Autodesk Fusion 360 part; units mm, degrees
(part 2 of 9)
  spline S7 degree 5 poles (-8.2602, -45.0085) (-8.2574, -44.9998) (-8.2518, -44.9823) (-8.2434, -44.9561) (-8.2325, -44.9211) (-8.2192, -44.8775) (-8.2062, -44.8338) (-8.1934, -44.7902) (-8.181, -44.7465) (-8.1689, -44.7029) (-8.1571, -44.6593) (-8.1456, -44.6157) (-8.1344, -44.5722) (-8.1235, -44.5286) (-8.1129, -44.4851) (-8.1026, -44.4416) (-8.0927, -44.3982) (-8.083, -44.3547) (-8.0737, -44.3113) (-8.0647, -44.268) (-8.056, -44.2247) (-8.0476, -44.1814) (-8.0396, -44.1381) (-8.0318, -44.0949) (-8.0244, -44.0518) (-8.0174, -44.0087) (-8.0106, -43.9656) (-8.0042, -43.9226) (-7.9981, -43.8797) (-7.9923, -43.8368) (-7.9869, -43.794) (-7.9818, -43.7512) (-7.9771, -43.7085) (-7.9727, -43.6659) (-7.9686, -43.6233) (-7.9649, -43.5808) (-7.9616, -43.5384) (-7.9585, -43.4961) (-7.9559, -43.4538) (-7.9536, -43.4116) (-7.9516, -43.3695) (-7.9501, -43.3275) (-7.9489, -43.2857) (-7.948, -43.2439) (-7.9476, -43.2022) (-7.9475, -43.1606) (-7.9478, -43.1191) (-7.9485, -43.0777) (-7.9495, -43.0364) (-7.951, -42.9953) (-7.9528, -42.9542) (-7.9551, -42.9133) (-7.9578, -42.8726) (-7.961, -42.832) (-7.9646, -42.7915) (-7.9686, -42.7512) (-7.9731, -42.7111) (-7.9779, -42.671) (-7.9831, -42.6312) (-7.9888, -42.5915) (-7.995, -42.552) (-8.0019, -42.5127) (-8.0095, -42.4737) (-8.0177, -42.435) (-8.0265, -42.3965) (-8.0358, -42.3583) (-8.0454, -42.3202) (-8.0554, -42.2822) (-8.0658, -42.2445) (-8.077, -42.2071) (-8.0895, -42.1703) (-8.1011, -42.1416) (-8.1108, -42.1205) (-8.1177, -42.1066) (-8.1213, -42.0998) knots -1 -1 -1 -1 -1 -1 -0.98571429 -0.97142857 -0.95714286 -0.94285714 -0.92857143 -0.91428571 -0.9 -0.88571429 -0.87142857 -0.85714286 -0.84285714 -0.82857143 -0.81428571 -0.8 -0.78571429 -0.77142857 -0.75714286 -0.74285714 -0.72857143 -0.71428571 -0.7 -0.68571429 -0.67142857 -0.65714286 -0.64285714 -0.62857143 -0.61428571 -0.6 -0.58571429 -0.57142857 -0.55714286 -0.54285714 -0.52857143 -0.51428571 -0.5 -0.48571429 -0.47142857 -0.45714286 -0.44285714 -0.42857143 -0.41428571 -0.4 -0.38571429 -0.37142857 -0.35714286 -0.34285714 -0.32857143 -0.31428571 -0.3 -0.28571429 -0.27142857 -0.25714286 -0.24285714 -0.22857143 -0.21428571 -0.2 -0.18571429 -0.17142857 -0.15714286 -0.14285714 -0.12857143 -0.11428571 -0.1 -0.08571429 -0.07142857 -0.05714286 -0.04285714 -0.02857143 -0.01428571 0 0 0 0 0 0
  line L7 (-8.1213, -42.0998) -> (-8.7529, -40.891)
  arc A15 (-8.5688, -40.2318) -> (-8.7529, -40.891) centre (-8.3098, -40.6595) ccw
  arc A16 (-8.5688, -40.2318) -> (-7.5487, -39.4906) centre (-12.4806, -33.7751) ccw
  arc A17 (-6.8649, -39.5193) -> (-7.5487, -39.4906) centre (-7.222, -39.8692) ccw
  line L8 (-6.8649, -39.5193) -> (-5.9105, -40.4935)
  spline S8 degree 5 poles (-5.9105, -40.4935) (-5.905, -40.499) (-5.894, -40.5099) (-5.8769, -40.5256) (-5.8532, -40.5455) (-5.8221, -40.5688) (-5.79, -40.591) (-5.7573, -40.6126) (-5.7243, -40.6338) (-5.691, -40.6547) (-5.6575, -40.6754) (-5.6236, -40.6956) (-5.5894, -40.7154) (-5.5546, -40.7347) (-5.5194, -40.7533) (-5.4838, -40.7714) (-5.4478, -40.7891) (-5.4115, -40.8064) (-5.3749, -40.8234) (-5.338, -40.84) (-5.301, -40.8563) (-5.2636, -40.8722) (-5.226, -40.8878) (-5.1881, -40.903) (-5.1499, -40.9178) (-5.1114, -40.9322) (-5.0728, -40.9463) (-5.0338, -40.9601) (-4.9947, -40.9735) (-4.9553, -40.9866) (-4.9157, -40.9994) (-4.8759, -41.0118) (-4.8359, -41.024) (-4.7957, -41.0358) (-4.7553, -41.0472) (-4.7146, -41.0584) (-4.6738, -41.0692) (-4.6328, -41.0798) (-4.5916, -41.09) (-4.5502, -41.0999) (-4.5087, -41.1095) (-4.4669, -41.1188) (-4.425, -41.1278) (-4.383, -41.1365) (-4.3407, -41.1449) (-4.2983, -41.1529) (-4.2557, -41.1607) (-4.213, -41.1682) (-4.1701, -41.1754) (-4.1271, -41.1823) (-4.0839, -41.1888) (-4.0406, -41.1951) (-3.9971, -41.2011) (-3.9535, -41.2068) (-3.9098, -41.2122) (-3.8659, -41.2174) (-3.8218, -41.2222) (-3.7777, -41.2267) (-3.7334, -41.231) (-3.689, -41.2349) (-3.6445, -41.2386) (-3.5998, -41.242) (-3.555, -41.2451) (-3.5102, -41.2479) (-3.4651, -41.2504) (-3.42, -41.2527) (-3.3748, -41.2546) (-3.3295, -41.2563) (-3.284, -41.2576) (-3.2385, -41.2587) (-3.1928, -41.2596) (-3.1562, -41.26) (-3.1287, -41.2602) (-3.1104, -41.2602) (-3.1012, -41.2603) knots 0 0 0 0 0 0 0.01428571 0.02857143 0.04285714 0.05714286 0.07142857 0.08571429 0.1 0.11428571 0.12857143 0.14285714 0.15714286 0.17142857 0.18571429 0.2 0.21428571 0.22857143 0.24285714 0.25714286 0.27142857 0.28571429 0.3 0.31428571 0.32857143 0.34285714 0.35714286 0.37142857 0.38571429 0.4 0.41428571 0.42857143 0.44285714 0.45714286 0.47142857 0.48571429 0.5 0.51428571 0.52857143 0.54285714 0.55714286 0.57142857 0.58571429 0.6 0.61428571 0.62857143 0.64285714 0.65714286 0.67142857 0.68571429 0.7 0.71428571 0.72857143 0.74285714 0.75714286 0.77142857 0.78571429 0.8 0.81428571 0.82857143 0.84285714 0.85714286 0.87142857 0.88571429 0.9 0.91428571 0.92857143 0.94285714 0.95714286 0.97142857 0.98571429 1 1 1 1 1 1
  arc A18 (-3.1012, -41.2603) -> (-2.4634, -40.3824) centre (-12.4806, -33.7751) ccw
  spline S9 degree 5 poles (-2.4634, -40.3824) (-2.4663, -40.3737) (-2.472, -40.3563) (-2.4807, -40.3302) (-2.4924, -40.2955) (-2.5073, -40.2523) (-2.5224, -40.2094) (-2.5377, -40.1666) (-2.5533, -40.124) (-2.5692, -40.0816) (-2.5852, -40.0393) (-2.6015, -39.9973) (-2.6181, -39.9555) (-2.6349, -39.9139) (-2.6519, -39.8724) (-2.6691, -39.8312) (-2.6866, -39.7902) (-2.7043, -39.7494) (-2.7223, -39.7088) (-2.7405, -39.6684) (-2.7589, -39.6283) (-2.7776, -39.5883) (-2.7965, -39.5486) (-2.8156, -39.5091) (-2.835, -39.4699) (-2.8546, -39.4308) (-2.8745, -39.392) (-2.8945, -39.3535) (-2.9149, -39.3152) (-2.9354, -39.2771) (-2.9562, -39.2392) (-2.9772, -39.2017) (-2.9985, -39.1643) (-3.02, -39.1272) (-3.0417, -39.0904) (-3.0637, -39.0539) (-3.0859, -39.0176) (-3.1084, -38.9816) (-3.131, -38.9458) (-3.154, -38.9103) (-3.1771, -38.8751) (-3.2005, -38.8402) (-3.2242, -38.8056) (-3.2481, -38.7713) (-3.2722, -38.7373) (-3.2966, -38.7036) (-3.3213, -38.6702) (-3.3461, -38.6372) (-3.3712, -38.6044) (-3.3966, -38.5719) (-3.4222, -38.5398) (-3.4481, -38.5081) (-3.4742, -38.4767) (-3.5007, -38.4458) (-3.5274, -38.4152) (-3.5543, -38.3849) (-3.5815, -38.355) (-3.609, -38.3255) (-3.6366, -38.2963) (-3.6646, -38.2675) (-3.6928, -38.2392) (-3.7215, -38.2115) (-3.7505, -38.1844) (-3.7799, -38.1579) (-3.8096, -38.132) (-3.8396, -38.1065) (-3.8698, -38.0813) (-3.9002, -38.0564) (-3.9308, -38.032) (-3.9618, -38.0084) (-3.9936, -37.986) (-4.0198, -37.9696) (-4.0401, -37.9582) (-4.0538, -37.9511) (-4.0608, -37.9476) knots -1 -1 -1 -1 -1 -1 -0.98571429 -0.97142857 -0.95714286 -0.94285714 -0.92857143 -0.91428571 -0.9 -0.88571429 -0.87142857 -0.85714286 -0.84285714 -0.82857143 -0.81428571 -0.8 -0.78571429 -0.77142857 -0.75714286 -0.74285714 -0.72857143 -0.71428571 -0.7 -0.68571429 -0.67142857 -0.65714286 -0.64285714 -0.62857143 -0.61428571 -0.6 -0.58571429 -0.57142857 -0.55714286 -0.54285714 -0.52857143 -0.51428571 -0.5 -0.48571429 -0.47142857 -0.45714286 -0.44285714 -0.42857143 -0.41428571 -0.4 -0.38571429 -0.37142857 -0.35714286 -0.34285714 -0.32857143 -0.31428571 -0.3 -0.28571429 -0.27142857 -0.25714286 -0.24285714 -0.22857143 -0.21428571 -0.2 -0.18571429 -0.17142857 -0.15714286 -0.14285714 -0.12857143 -0.11428571 -0.1 -0.08571429 -0.07142857 -0.05714286 -0.04285714 -0.02857143 -0.01428571 0 0 0 0 0 0
  line L9 (-4.0608, -37.9476) -> (-5.2822, -37.341)
  arc A19 (-5.5208, -36.6995) -> (-5.2822, -37.341) centre (-5.0598, -36.8932) ccw
  arc A20 (-5.5208, -36.6995) -> (-5.1311, -35.5002) centre (-12.4806, -33.7751) ccw
  arc A21 (-4.561, -35.1214) -> (-5.1311, -35.5002) centre (-4.6443, -35.6144) ccw
  line L10 (-4.561, -35.1214) -> (-3.2163, -35.3486)
  spline S10 degree 5 poles (-3.2163, -35.3486) (-3.2087, -35.3499) (-3.1933, -35.3522) (-3.1703, -35.3549) (-3.1394, -35.357) (-3.1005, -35.3576) (-3.0615, -35.3567) (-3.0224, -35.3549) (-2.9832, -35.3527) (-2.944, -35.35) (-2.9048, -35.347) (-2.8654, -35.3435) (-2.8261, -35.3394) (-2.7867, -35.3345) (-2.7472, -35.3289) (-2.7077, -35.3227) (-2.6682, -35.3158) (-2.6287, -35.3085) (-2.5891, -35.3007) (-2.5495, -35.2925) (-2.51, -35.2838) (-2.4704, -35.2748) (-2.4308, -35.2653) (-2.3912, -35.2553) (-2.3516, -35.2448) (-2.312, -35.2339) (-2.2724, -35.2225) (-2.2328, -35.2108) (-2.1933, -35.1986) (-2.1537, -35.1861) (-2.1142, -35.1732) (-2.0747, -35.1599) (-2.0352, -35.1462) (-1.9957, -35.1321) (-1.9562, -35.1176) (-1.9168, -35.1027) (-1.8774, -35.0875) (-1.838, -35.0719) (-1.7987, -35.056) (-1.7594, -35.0397) (-1.7201, -35.023) (-1.6809, -35.006) (-1.6417, -34.9886) (-1.6026, -34.9709) (-1.5635, -34.9529) (-1.5244, -34.9345) (-1.4854, -34.9158) (-1.4464, -34.8967) (-1.4075, -34.8773) (-1.3687, -34.8576) (-1.3299, -34.8375) (-1.2911, -34.8171) (-1.2524, -34.7964) (-1.2138, -34.7754) (-1.1752, -34.7541) (-1.1367, -34.7324) (-1.0982, -34.7105) (-1.0599, -34.6882) (-1.0215, -34.6656) (-0.9833, -34.6427) (-0.9451, -34.6195) (-0.907, -34.596) (-0.8689, -34.5722) (-0.831, -34.548) (-0.7931, -34.5236) (-0.7553, -34.4989) (-0.7175, -34.4739) (-0.6799, -34.4486) (-0.6423, -34.423) (-0.6048, -34.3971) (-0.5674, -34.371) (-0.5375, -34.3498) (-0.5152, -34.3338) (-0.5003, -34.3231) (-0.4928, -34.3177) knots 0 0 0 0 0 0 0.01428571 0.02857143 0.04285714 0.05714286 0.07142857 0.08571429 0.1 0.11428571 0.12857143 0.14285714 0.15714286 0.17142857 0.18571429 0.2 0.21428571 0.22857143 0.24285714 0.25714286 0.27142857 0.28571429 0.3 0.31428571 0.32857143 0.34285714 0.35714286 0.37142857 0.38571429 0.4 0.41428571 0.42857143 0.44285714 0.45714286 0.47142857 0.48571429 0.5 0.51428571 0.52857143 0.54285714 0.55714286 0.57142857 0.58571429 0.6 0.61428571 0.62857143 0.64285714 0.65714286 0.67142857 0.68571429 0.7 0.71428571 0.72857143 0.74285714 0.75714286 0.77142857 0.78571429 0.8 0.81428571 0.82857143 0.84285714 0.85714286 0.87142857 0.88571429 0.9 0.91428571 0.92857143 0.94285714 0.95714286 0.97142857 0.98571429 1 1 1 1 1 1
  arc A22 (-0.4928, -34.3177) -> (-0.4928, -33.2326) centre (-12.4806, -33.7751) ccw
  spline S11 degree 5 poles (-0.4928, -33.2326) (-0.5003, -33.2272) (-0.5152, -33.2165) (-0.5375, -33.2005) (-0.5674, -33.1793) (-0.6048, -33.1532) (-0.6423, -33.1273) (-0.6799, -33.1017) (-0.7175, -33.0764) (-0.7553, -33.0514) (-0.7931, -33.0267) (-0.831, -33.0022) (-0.8689, -32.9781) (-0.907, -32.9543) (-0.9451, -32.9308) (-0.9833, -32.9076) (-1.0215, -32.8847) (-1.0599, -32.8621) (-1.0982, -32.8398) (-1.1367, -32.8179) (-1.1752, -32.7962) (-1.2138, -32.7749) (-1.2524, -32.7538) (-1.2911, -32.7331) (-1.3299, -32.7128) (-1.3687, -32.6927) (-1.4075, -32.673) (-1.4464, -32.6536) (-1.4854, -32.6345) (-1.5244, -32.6158) (-1.5635, -32.5974) (-1.6026, -32.5794) (-1.6417, -32.5617) (-1.6809, -32.5443) (-1.7201, -32.5273) (-1.7594, -32.5106) (-1.7987, -32.4943) (-1.838, -32.4784) (-1.8774, -32.4628) (-1.9168, -32.4476) (-1.9562, -32.4327) (-1.9957, -32.4182) (-2.0352, -32.4041) (-2.0747, -32.3904) (-2.1142, -32.3771) (-2.1537, -32.3642) (-2.1933, -32.3517) (-2.2328, -32.3395) (-2.2724, -32.3277) (-2.312, -32.3164) (-2.3516, -32.3055) (-2.3912, -32.295) (-2.4308, -32.285) (-2.4704, -32.2755) (-2.51, -32.2664) (-2.5495, -32.2578) (-2.5891, -32.2496) (-2.6287, -32.2418) (-2.6682, -32.2345) (-2.7077, -32.2276) (-2.7472, -32.2213) (-2.7867, -32.2157) (-2.8261, -32.2109) (-2.8654, -32.2067) (-2.9048, -32.2033) (-2.944, -32.2003) (-2.9832, -32.1976) (-3.0224, -32.1954) (-3.0615, -32.1936) (-3.1005, -32.1927) (-3.1394, -32.1933) (-3.1703, -32.1954) (-3.1933, -32.1981) (-3.2087, -32.2004) (-3.2163, -32.2017) knots -1 -1 -1 -1 -1 -1 -0.98571429 -0.97142857 -0.95714286 -0.94285714 -0.92857143 -0.91428571 -0.9 -0.88571429 -0.87142857 -0.85714286 -0.84285714 -0.82857143 -0.81428571 -0.8 -0.78571429 -0.77142857 -0.75714286 -0.74285714 -0.72857143 -0.71428571 -0.7 -0.68571429 -0.67142857 -0.65714286 -0.64285714 -0.62857143 -0.61428571 -0.6 -0.58571429 -0.57142857 -0.55714286 -0.54285714 -0.52857143 -0.51428571 -0.5 -0.48571429 -0.47142857 -0.45714286 -0.44285714 -0.42857143 -0.41428571 -0.4 -0.38571429 -0.37142857 -0.35714286 -0.34285714 -0.32857143 -0.31428571 -0.3 -0.28571429 -0.27142857 -0.25714286 -0.24285714 -0.22857143 -0.21428571 -0.2 -0.18571429 -0.17142857 -0.15714286 -0.14285714 -0.12857143 -0.11428571 -0.1 -0.08571429 -0.07142857 -0.05714286 -0.04285714 -0.02857143 -0.01428571 0 0 0 0 0 0
  line L11 (-3.2163, -32.2017) -> (-4.561, -32.4289)
  arc A23 (-5.1311, -32.0501) -> (-4.561, -32.4289) centre (-4.6443, -31.9359) ccw
  arc A24 (-5.1311, -32.0501) -> (-5.5208, -30.8508) centre (-12.4806, -33.7751) ccw
  arc A25 (-5.2822, -30.2093) -> (-5.5208, -30.8508) centre (-5.0598, -30.6571) ccw
  line L12 (-5.2822, -30.2093) -> (-4.0608, -29.6027)
  spline S12 degree 5 poles (-4.0608, -29.6027) (-4.0538, -29.5992) (-4.0401, -29.5921) (-4.0198, -29.5807) (-3.9936, -29.5643) (-3.9618, -29.5419) (-3.9308, -29.5183) (-3.9002, -29.4939) (-3.8698, -29.469) (-3.8396, -29.4438) (-3.8096, -29.4183) (-3.7799, -29.3924) (-3.7505, -29.3659) (-3.7215, -29.3388) (-3.6928, -29.3111) (-3.6646, -29.2828) (-3.6366, -29.254) (-3.609, -29.2248) (-3.5815, -29.1953) (-3.5543, -29.1654) (-3.5274, -29.1351) (-3.5007, -29.1045) (-3.4742, -29.0736) (-3.4481, -29.0422) (-3.4222, -29.0105) (-3.3966, -28.9784) (-3.3712, -28.9459) (-3.3461, -28.9131) (-3.3213, -28.8801) (-3.2966, -28.8467) (-3.2722, -28.813) (-3.2481, -28.779) (-3.2242, -28.7447) (-3.2005, -28.7101) (-3.1771, -28.6752) (-3.154, -28.64) (-3.131, -28.6045) (-3.1084, -28.5687) (-3.0859, -28.5327) (-3.0637, -28.4964) (-3.0417, -28.4599) (-3.02, -28.423) (-2.9985, -28.386) (-2.9772, -28.3486) (-2.9562, -28.311) (-2.9354, -28.2732) (-2.9149, -28.2351) (-2.8945, -28.1968) (-2.8745, -28.1582) (-2.8546, -28.1194) (-2.835, -28.0804) (-2.8156, -28.0411) (-2.7965, -28.0017) (-2.7776, -27.9619) (-2.7589, -27.922) (-2.7405, -27.8818) (-2.7223, -27.8415) (-2.7043, -27.8009) (-2.6866, -27.7601) (-2.6691, -27.7191) (-2.6519, -27.6779) (-2.6349, -27.6364) (-2.6181, -27.5948) (-2.6015, -27.553) (-2.5852, -27.511) (-2.5692, -27.4687) (-2.5533, -27.4263) (-2.5377, -27.3837) (-2.5224, -27.3409) (-2.5073, -27.2979) (-2.4924, -27.2548) (-2.4807, -27.2201) (-2.472, -27.194) (-2.4663, -27.1766) (-2.4634, -27.1678) knots 0 0 0 0 0 0 0.01428571 0.02857143 0.04285714 0.05714286 0.07142857 0.08571429 0.1 0.11428571 0.12857143 0.14285714 0.15714286 0.17142857 0.18571429 0.2 0.21428571 0.22857143 0.24285714 0.25714286 0.27142857 0.28571429 0.3 0.31428571 0.32857143 0.34285714 0.35714286 0.37142857 0.38571429 0.4 0.41428571 0.42857143 0.44285714 0.45714286 0.47142857 0.48571429 0.5 0.51428571 0.52857143 0.54285714 0.55714286 0.57142857 0.58571429 0.6 0.61428571 0.62857143 0.64285714 0.65714286 0.67142857 0.68571429 0.7 0.71428571 0.72857143 0.74285714 0.75714286 0.77142857 0.78571429 0.8 0.81428571 0.82857143 0.84285714 0.85714286 0.87142857 0.88571429 0.9 0.91428571 0.92857143 0.94285714 0.95714286 0.97142857 0.98571429 1 1 1 1 1 1
  arc A26 (-2.4634, -27.1678) -> (-3.1012, -26.29) centre (-12.4806, -33.7751) ccw
  spline S13 degree 5 poles (-3.1012, -26.29) (-3.1104, -26.29) (-3.1287, -26.2901) (-3.1562, -26.2903) (-3.1928, -26.2907) (-3.2385, -26.2915) (-3.284, -26.2926) (-3.3295, -26.294) (-3.3748, -26.2957) (-3.42, -26.2976) (-3.4651, -26.2999) (-3.5102, -26.3024) (-3.555, -26.3052) (-3.5998, -26.3083) (-3.6445, -26.3117) (-3.689, -26.3153) (-3.7334, -26.3193) (-3.7777, -26.3236) (-3.8218, -26.3281) (-3.8659, -26.3329) (-3.9098, -26.338) (-3.9535, -26.3435) (-3.9971, -26.3492) (-4.0406, -26.3552) (-4.0839, -26.3614) (-4.1271, -26.368) (-4.1701, -26.3749) (-4.213, -26.3821) (-4.2557, -26.3896) (-4.2983, -26.3974) (-4.3407, -26.4054) (-4.383, -26.4138) (-4.425, -26.4225) (-4.4669, -26.4315) (-4.5087, -26.4408) (-4.5502, -26.4504) (-4.5916, -26.4603) (-4.6328, -26.4705) (-4.6738, -26.481) (-4.7146, -26.4919) (-4.7553, -26.503) (-4.7957, -26.5145) (-4.8359, -26.5263) (-4.8759, -26.5384) (-4.9157, -26.5509) (-4.9553, -26.5637) (-4.9947, -26.5768) (-5.0338, -26.5902) (-5.0728, -26.604) (-5.1114, -26.6181) (-5.1499, -26.6325) (-5.1881, -26.6473) (-5.226, -26.6625) (-5.2636, -26.6781) (-5.301, -26.694) (-5.338, -26.7103) (-5.3749, -26.7269) (-5.4115, -26.7439) (-5.4478, -26.7612) (-5.4838, -26.7788) (-5.5194, -26.797) (-5.5546, -26.8156) (-5.5894, -26.8349) (-5.6236, -26.8547) (-5.6575, -26.8749) (-5.691, -26.8956) (-5.7243, -26.9165) (-5.7573, -26.9377) (-5.79, -26.9592) (-5.8221, -26.9815) (-5.8532, -27.0048) (-5.8769, -27.0246) (-5.894, -27.0404) (-5.905, -27.0513) (-5.9105, -27.0568) knots -1 -1 -1 -1 -1 -1 -0.98571429 -0.97142857 -0.95714286 -0.94285714 -0.92857143 -0.91428571 -0.9 -0.88571429 -0.87142857 -0.85714286 -0.84285714 -0.82857143 -0.81428571 -0.8 -0.78571429 -0.77142857 -0.75714286 -0.74285714 -0.72857143 -0.71428571 -0.7 -0.68571429 -0.67142857 -0.65714286 -0.64285714 -0.62857143 -0.61428571 -0.6 -0.58571429 -0.57142857 -0.55714286 -0.54285714 -0.52857143 -0.51428571 -0.5 -0.48571429 -0.47142857 -0.45714286 -0.44285714 -0.42857143 -0.41428571 -0.4 -0.38571429 -0.37142857 -0.35714286 -0.34285714 -0.32857143 -0.31428571 -0.3 -0.28571429 -0.27142857 -0.25714286 -0.24285714 -0.22857143 -0.21428571 -0.2 -0.18571429 -0.17142857 -0.15714286 -0.14285714 -0.12857143 -0.11428571 -0.1 -0.08571429 -0.07142857 -0.05714286 -0.04285714 -0.02857143 -0.01428571 0 0 0 0 0 0
  line L13 (-5.9105, -27.0568) -> (-6.8649, -28.031)
  arc A27 (-7.5487, -28.0597) -> (-6.8649, -28.031) centre (-7.222, -27.6811) ccw
  arc A28 (-7.5487, -28.0597) -> (-8.5688, -27.3185) centre (-12.4806, -33.7751) ccw
  arc A29 (-8.7529, -26.6593) -> (-8.5688, -27.3185) centre (-8.3098, -26.8908) ccw
  line L14 (-8.7529, -26.6593) -> (-8.1213, -25.4505)
  spline S14 degree 5 poles (-8.1213, -25.4505) (-8.1177, -25.4437) (-8.1108, -25.4298) (-8.1011, -25.4087) (-8.0895, -25.3799) (-8.077, -25.3432) (-8.0658, -25.3058) (-8.0554, -25.2681) (-8.0454, -25.2301) (-8.0358, -25.192) (-8.0265, -25.1537) (-8.0177, -25.1153) (-8.0095, -25.0766) (-8.0019, -25.0376) (-7.995, -24.9983) (-7.9888, -24.9588) (-7.9831, -24.9191) (-7.9779, -24.8792) (-7.9731, -24.8392) (-7.9686, -24.799) (-7.9646, -24.7587) (-7.961, -24.7183) (-7.9578, -24.6777) (-7.9551, -24.637) (-7.9528, -24.5961) (-7.951, -24.555) (-7.9495, -24.5139) (-7.9485, -24.4726) (-7.9478, -24.4312) (-7.9475, -24.3897) (-7.9476, -24.3481) (-7.948, -24.3064) (-7.9489, -24.2646) (-7.9501, -24.2227) (-7.9516, -24.1807) (-7.9536, -24.1387) (-7.9559, -24.0965) (-7.9585, -24.0542) (-7.9616, -24.0119) (-7.9649, -23.9695) (-7.9686, -23.927) (-7.9727, -23.8844) (-7.9771, -23.8418) (-7.9818, -23.7991) (-7.9869, -23.7563) (-7.9923, -23.7135) (-7.9981, -23.6706) (-8.0042, -23.6276) (-8.0106, -23.5846) (-8.0174, -23.5416) (-8.0244, -23.4985) (-8.0318, -23.4553) (-8.0396, -23.4121) (-8.0476, -23.3689) (-8.056, -23.3256) (-8.0647, -23.2823) (-8.0737, -23.2389) (-8.083, -23.1956) (-8.0927, -23.1521) (-8.1026, -23.1087) (-8.1129, -23.0652) (-8.1235, -23.0217) (-8.1344, -22.9781) (-8.1456, -22.9346) (-8.1571, -22.891) (-8.1689, -22.8474) (-8.181, -22.8038) (-8.1934, -22.7601) (-8.2062, -22.7165) (-8.2192, -22.6728) (-8.2325, -22.6292) (-8.2434, -22.5942) (-8.2518, -22.568) (-8.2574, -22.5505) (-8.2602, -22.5418) knots 0 0 0 0 0 0 0.01428571 0.02857143 0.04285714 0.05714286 0.07142857 0.08571429 0.1 0.11428571 0.12857143 0.14285714 0.15714286 0.17142857 0.18571429 0.2 0.21428571 0.22857143 0.24285714 0.25714286 0.27142857 0.28571429 0.3 0.31428571 0.32857143 0.34285714 0.35714286 0.37142857 0.38571429 0.4 0.41428571 0.42857143 0.44285714 0.45714286 0.47142857 0.48571429 0.5 0.51428571 0.52857143 0.54285714 0.55714286 0.57142857 0.58571429 0.6 0.61428571 0.62857143 0.64285714 0.65714286 0.67142857 0.68571429 0.7 0.71428571 0.72857143 0.74285714 0.75714286 0.77142857 0.78571429 0.8 0.81428571 0.82857143 0.84285714 0.85714286 0.87142857 0.88571429 0.9 0.91428571 0.92857143 0.94285714 0.95714286 0.97142857 0.98571429 1 1 1 1 1 1
  arc A30 (-8.2602, -22.5418) -> (-9.2921, -22.2065) centre (-12.4806, -33.7751) ccw
  spline S15 degree 5 poles (-9.2921, -22.2065) (-9.2995, -22.2119) (-9.3144, -22.2227) (-9.3365, -22.2391) (-9.3658, -22.2609) (-9.4023, -22.2884) (-9.4385, -22.3161) (-9.4745, -22.3439) (-9.5102, -22.3719) (-9.5456, -22.4001) (-9.5808, -22.4284) (-9.6157, -22.4569) (-9.6504, -22.4855) (-9.6848, -22.5144) (-9.7189, -22.5433) (-9.7528, -22.5725) (-9.7864, -22.6018) (-9.8197, -22.6313) (-9.8528, -22.6609) (-9.8856, -22.6907) (-9.9181, -22.7206) (-9.9503, -22.7507) (-9.9822, -22.7809) (-10.0138, -22.8113) (-10.0452, -22.8419) (-10.0763, -22.8726) (-10.107, -22.9035) (-10.1375, -22.9345) (-10.1677, -22.9657) (-10.1975, -22.997) (-10.2271, -23.0284) (-10.2563, -23.06) (-10.2853, -23.0918) (-10.3139, -23.1237) (-10.3422, -23.1558) (-10.3702, -23.188) (-10.3978, -23.2203) (-10.4251, -23.2528) (-10.4521, -23.2854) (-10.4788, -23.3182) (-10.5051, -23.3511) (-10.5311, -23.3841) (-10.5567, -23.4173) (-10.5819, -23.4506) (-10.6068, -23.4841) (-10.6313, -23.5177) (-10.6554, -23.5515) (-10.6792, -23.5853) (-10.7026, -23.6193) (-10.7257, -23.6535) (-10.7483, -23.6878) (-10.7705, -23.7222) (-10.7922, -23.7568) (-10.8135, -23.7915) (-10.8343, -23.8263) (-10.8548, -23.8613) (-10.8748, -23.8964) (-10.8944, -23.9316) (-10.9136, -23.9669) (-10.9324, -24.0024) (-10.9505, -24.038) (-10.9681, -24.0738) (-10.9849, -24.1098) (-11.001, -24.146) (-11.0164, -24.1823) (-11.0314, -24.2187) (-11.046, -24.2552) (-11.0603, -24.2917) (-11.0741, -24.3284) (-11.087, -24.3652) (-11.0984, -24.4023) (-11.106, -24.4323) (-11.1105, -24.4551) (-11.113, -24.4704) (-11.1142, -24.4781) knots -1 -1 -1 -1 -1 -1 -0.98571429 -0.97142857 -0.95714286 -0.94285714 -0.92857143 -0.91428571 -0.9 -0.88571429 -0.87142857 -0.85714286 -0.84285714 -0.82857143 -0.81428571 -0.8 -0.78571429 -0.77142857 -0.75714286 -0.74285714 -0.72857143 -0.71428571 -0.7 -0.68571429 -0.67142857 -0.65714286 -0.64285714 -0.62857143 -0.61428571 -0.6 -0.58571429 -0.57142857 -0.55714286 -0.54285714 -0.52857143 -0.51428571 -0.5 -0.48571429 -0.47142857 -0.45714286 -0.44285714 -0.42857143 -0.41428571 -0.4 -0.38571429 -0.37142857 -0.35714286 -0.34285714 -0.32857143 -0.31428571 -0.3 -0.28571429 -0.27142857 -0.25714286 -0.24285714 -0.22857143 -0.21428571 -0.2 -0.18571429 -0.17142857 -0.15714286 -0.14285714 -0.12857143 -0.11428571 -0.1 -0.08571429 -0.07142857 -0.05714286 -0.04285714 -0.02857143 -0.01428571 0 0 0 0 0 0
  line L15 (-11.1142, -24.4781) -> (-11.3137, -25.8272)
  arc A31 (-11.8501, -26.2523) -> (-11.3137, -25.8272) centre (-11.8083, -25.7541) ccw
  arc A32 (-11.8501, -26.2523) -> (-13.1111, -26.2523) centre (-12.4806, -33.7751) ccw
  arc A33 (-13.6474, -25.8272) -> (-13.1111, -26.2523) centre (-13.1528, -25.7541) ccw
  line L16 (-13.6474, -25.8272) -> (-13.847, -24.4781)
  spline S16 degree 5 poles (-13.847, -24.4781) (-13.8481, -24.4704) (-13.8506, -24.4551) (-13.8552, -24.4323) (-13.8627, -24.4023) (-13.8742, -24.3652) (-13.887, -24.3284) (-13.9008, -24.2917) (-13.9151, -24.2552) (-13.9297, -24.2187) (-13.9447, -24.1823) (-13.9602, -24.146) (-13.9763, -24.1098) (-13.9931, -24.0738) (-14.0106, -24.038) (-14.0288, -24.0024) (-14.0475, -23.9669) (-14.0667, -23.9316) (-14.0863, -23.8964) (-14.1064, -23.8613) (-14.1268, -23.8263) (-14.1476, -23.7915) (-14.1689, -23.7568) (-14.1907, -23.7222) (-14.2129, -23.6878) (-14.2355, -23.6535) (-14.2585, -23.6193) (-14.2819, -23.5853) (-14.3057, -23.5515) (-14.3298, -23.5177) (-14.3544, -23.4841) (-14.3792, -23.4506) (-14.4045, -23.4173) (-14.4301, -23.3841) (-14.456, -23.3511) (-14.4823, -23.3182) (-14.509, -23.2854) (-14.536, -23.2528) (-14.5633, -23.2203) (-14.591, -23.188) (-14.6189, -23.1558) (-14.6472, -23.1237) (-14.6759, -23.0918) (-14.7048, -23.06) (-14.734, -23.0284) (-14.7636, -22.997) (-14.7935, -22.9657) (-14.8236, -22.9345) (-14.8541, -22.9035) (-14.8849, -22.8726) (-14.9159, -22.8419) (-14.9473, -22.8113) (-14.9789, -22.7809) (-15.0109, -22.7507) (-15.0431, -22.7206) (-15.0756, -22.6907) (-15.1084, -22.6609) (-15.1414, -22.6313) (-15.1747, -22.6018) (-15.2083, -22.5725) (-15.2422, -22.5433) (-15.2763, -22.5144) (-15.3107, -22.4855) (-15.3454, -22.4569) (-15.3803, -22.4284) (-15.4155, -22.4001) (-15.451, -22.3719) (-15.4867, -22.3439) (-15.5226, -22.3161) (-15.5588, -22.2884) (-15.5953, -22.2609) (-15.6246, -22.2391) (-15.6468, -22.2227) (-15.6616, -22.2119) (-15.669, -22.2065) knots 0 0 0 0 0 0 0.01428571 0.02857143 0.04285714 0.05714286 0.07142857 0.08571429 0.1 0.11428571 0.12857143 0.14285714 0.15714286 0.17142857 0.18571429 0.2 0.21428571 0.22857143 0.24285714 0.25714286 0.27142857 0.28571429 0.3 0.31428571 0.32857143 0.34285714 0.35714286 0.37142857 0.38571429 0.4 0.41428571 0.42857143 0.44285714 0.45714286 0.47142857 0.48571429 0.5 0.51428571 0.52857143 0.54285714 0.55714286 0.57142857 0.58571429 0.6 0.61428571 0.62857143 0.64285714 0.65714286 0.67142857 0.68571429 0.7 0.71428571 0.72857143 0.74285714 0.75714286 0.77142857 0.78571429 0.8 0.81428571 0.82857143 0.84285714 0.85714286 0.87142857 0.88571429 0.9 0.91428571 0.92857143 0.94285714 0.95714286 0.97142857 0.98571429 1 1 1 1 1 1
  arc A34 (-15.669, -22.2065) -> (-16.701, -22.5418) centre (-12.4806, -33.7751) ccw
  spline S17 degree 5 poles (-16.701, -22.5418) (-16.7038, -22.5505) (-16.7094, -22.568) (-16.7177, -22.5942) (-16.7286, -22.6292) (-16.7419, -22.6728) (-16.755, -22.7165) (-16.7677, -22.7601) (-16.7801, -22.8038) (-16.7922, -22.8474) (-16.8041, -22.891) (-16.8156, -22.9346) (-16.8268, -22.9781) (-16.8377, -23.0217) (-16.8482, -23.0652) (-16.8585, -23.1087) (-16.8685, -23.1521) (-16.8781, -23.1956) (-16.8874, -23.2389) (-16.8965, -23.2823) (-16.9051, -23.3256) (-16.9135, -23.3689) (-16.9216, -23.4121) (-16.9293, -23.4553) (-16.9367, -23.4985) (-16.9438, -23.5416) (-16.9505, -23.5846) (-16.957, -23.6276) (-16.963, -23.6706) (-16.9688, -23.7135) (-16.9742, -23.7563) (-16.9793, -23.7991) (-16.984, -23.8418) (-16.9884, -23.8844) (-16.9925, -23.927) (-16.9962, -23.9695) (-16.9996, -24.0119) (-17.0026, -24.0542) (-17.0053, -24.0965) (-17.0076, -24.1387) (-17.0095, -24.1807) (-17.0111, -24.2227) (-17.0123, -24.2646) (-17.0131, -24.3064) (-17.0136, -24.3481) (-17.0136, -24.3897) (-17.0133, -24.4312) (-17.0127, -24.4726) (-17.0116, -24.5139) (-17.0102, -24.555) (-17.0083, -24.5961) (-17.006, -24.637) (-17.0033, -24.6777) (-17.0001, -24.7183) (-16.9965, -24.7587) (-16.9925, -24.799) (-16.9881, -24.8392) (-16.9832, -24.8792) (-16.978, -24.9191) (-16.9723, -24.9588) (-16.9661, -24.9983) (-16.9592, -25.0376) (-16.9517, -25.0766) (-16.9434, -25.1153) (-16.9346, -25.1537) (-16.9253, -25.192) (-16.9157, -25.2301) (-16.9058, -25.2681) (-16.8954, -25.3058) (-16.8842, -25.3432) (-16.8716, -25.3799) (-16.86, -25.4087) (-16.8503, -25.4298) (-16.8434, -25.4437) (-16.8398, -25.4505) knots -1 -1 -1 -1 -1 -1 -0.98571429 -0.97142857 -0.95714286 -0.94285714 -0.92857143 -0.91428571 -0.9 -0.88571429 -0.87142857 -0.85714286 -0.84285714 -0.82857143 -0.81428571 -0.8 -0.78571429 -0.77142857 -0.75714286 -0.74285714 -0.72857143 -0.71428571 -0.7 -0.68571429 -0.67142857 -0.65714286 -0.64285714 -0.62857143 -0.61428571 -0.6 -0.58571429 -0.57142857 -0.55714286 -0.54285714 -0.52857143 -0.51428571 -0.5 -0.48571429 -0.47142857 -0.45714286 -0.44285714 -0.42857143 -0.41428571 -0.4 -0.38571429 -0.37142857 -0.35714286 -0.34285714 -0.32857143 -0.31428571 -0.3 -0.28571429 -0.27142857 -0.25714286 -0.24285714 -0.22857143 -0.21428571 -0.2 -0.18571429 -0.17142857 -0.15714286 -0.14285714 -0.12857143 -0.11428571 -0.1 -0.08571429 -0.07142857 -0.05714286 -0.04285714 -0.02857143 -0.01428571 0 0 0 0 0 0
  line L17 (-16.8398, -25.4505) -> (-16.2082, -26.6593)
  arc A35 (-16.3923, -27.3185) -> (-16.2082, -26.6593) centre (-16.6514, -26.8908) ccw
  arc A36 (-16.3923, -27.3185) -> (-17.4125, -28.0597) centre (-12.4806, -33.7751) ccw
  arc A37 (-18.0963, -28.031) -> (-17.4125, -28.0597) centre (-17.7391, -27.6811) ccw
  line L18 (-18.0963, -28.031) -> (-19.0507, -27.0568)
  spline S18 degree 5 poles (-19.0507, -27.0568) (-19.0561, -27.0513) (-19.0671, -27.0404) (-19.0842, -27.0246) (-19.108, -27.0048) (-19.139, -26.9815) (-19.1711, -26.9592) (-19.2038, -26.9377) (-19.2368, -26.9165) (-19.2701, -26.8956) (-19.3036, -26.8749) (-19.3375, -26.8547) (-19.3718, -26.8349) (-19.4065, -26.8156) (-19.4417, -26.797) (-19.4773, -26.7788) (-19.5134, -26.7612) (-19.5497, -26.7439) (-19.5863, -26.7269) (-19.6231, -26.7103) (-19.6602, -26.694) (-19.6975, -26.6781) (-19.7351, -26.6625) (-19.7731, -26.6473) (-19.8112, -26.6325) (-19.8497, -26.6181) (-19.8884, -26.604) (-19.9273, -26.5902) (-19.9665, -26.5768) (-20.0058, -26.5637) (-20.0454, -26.5509) (-20.0852, -26.5384) (-20.1252, -26.5263) (-20.1654, -26.5145) (-20.2059, -26.503) (-20.2465, -26.4919) (-20.2873, -26.481) (-20.3283, -26.4705) (-20.3695, -26.4603) (-20.4109, -26.4504) (-20.4525, -26.4408) (-20.4942, -26.4315) (-20.5361, -26.4225) (-20.5782, -26.4138) (-20.6204, -26.4054) (-20.6628, -26.3974) (-20.7054, -26.3896) (-20.7481, -26.3821) (-20.791, -26.3749) (-20.834, -26.368) (-20.8772, -26.3614) (-20.9205, -26.3552) (-20.964, -26.3492) (-21.0076, -26.3435) (-21.0514, -26.338) (-21.0953, -26.3329) (-21.1393, -26.3281) (-21.1834, -26.3236) (-21.2277, -26.3193) (-21.2721, -26.3153) (-21.3167, -26.3117) (-21.3613, -26.3083) (-21.4061, -26.3052) (-21.451, -26.3024) (-21.496, -26.2999) (-21.5411, -26.2976) (-21.5863, -26.2957) (-21.6317, -26.294) (-21.6771, -26.2926) (-21.7227, -26.2915) (-21.7683, -26.2907) (-21.8049, -26.2903) (-21.8324, -26.2901) (-21.8508, -26.29) (-21.86, -26.29) knots 0 0 0 0 0 0 0.01428571 0.02857143 0.04285714 0.05714286 0.07142857 0.08571429 0.1 0.11428571 0.12857143 0.14285714 0.15714286 0.17142857 0.18571429 0.2 0.21428571 0.22857143 0.24285714 0.25714286 0.27142857 0.28571429 0.3 0.31428571 0.32857143 0.34285714 0.35714286 0.37142857 0.38571429 0.4 0.41428571 0.42857143 0.44285714 0.45714286 0.47142857 0.48571429 0.5 0.51428571 0.52857143 0.54285714 0.55714286 0.57142857 0.58571429 0.6 0.61428571 0.62857143 0.64285714 0.65714286 0.67142857 0.68571429 0.7 0.71428571 0.72857143 0.74285714 0.75714286 0.77142857 0.78571429 0.8 0.81428571 0.82857143 0.84285714 0.85714286 0.87142857 0.88571429 0.9 0.91428571 0.92857143 0.94285714 0.95714286 0.97142857 0.98571429 1 1 1 1 1 1
  arc A38 (-21.86, -26.29) -> (-22.4977, -27.1678) centre (-12.4806, -33.7751) ccw
  spline S19 degree 5 poles (-22.4977, -27.1678) (-22.4949, -27.1766) (-22.4891, -27.194) (-22.4805, -27.2201) (-22.4687, -27.2548) (-22.4539, -27.2979) (-22.4387, -27.3409) (-22.4234, -27.3837) (-22.4078, -27.4263) (-22.392, -27.4687) (-22.3759, -27.511) (-22.3596, -27.553) (-22.343, -27.5948) (-22.3263, -27.6364) (-22.3092, -27.6779) (-22.292, -27.7191) (-22.2745, -27.7601) (-22.2568, -27.8009) (-22.2388, -27.8415) (-22.2206, -27.8818) (-22.2022, -27.922) (-22.1835, -27.9619) (-22.1646, -28.0017) (-22.1455, -28.0411) (-22.1261, -28.0804) (-22.1065, -28.1194) (-22.0867, -28.1582) (-22.0666, -28.1968) (-22.0463, -28.2351) (-22.0257, -28.2732) (-22.0049, -28.311) (-21.9839, -28.3486) (-21.9626, -28.386) (-21.9411, -28.423) (-21.9194, -28.4599) (-21.8974, -28.4964) (-21.8752, -28.5327) (-21.8528, -28.5687) (-21.8301, -28.6045) (-21.8072, -28.64) (-21.784, -28.6752) (-21.7606, -28.7101) (-21.7369, -28.7447) (-21.713, -28.779) (-21.6889, -28.813) (-21.6645, -28.8467) (-21.6399, -28.8801) (-21.615, -28.9131) (-21.5899, -28.9459) (-21.5645, -28.9784) (-21.5389, -29.0105) (-21.513, -29.0422) (-21.4869, -29.0736) (-21.4605, -29.1045) (-21.4338, -29.1351) (-21.4068, -29.1654) (-21.3796, -29.1953) (-21.3522, -29.2248) (-21.3245, -29.254) (-21.2966, -29.2828) (-21.2683, -29.3111) (-21.2397, -29.3388) (-21.2107, -29.3659) (-21.1812, -29.3924) (-21.1515, -29.4183) (-21.1215, -29.4438) (-21.0913, -29.469) (-21.061, -29.4939) (-21.0304, -29.5183) (-20.9993, -29.5419) (-20.9676, -29.5643) (-20.9413, -29.5807) (-20.9211, -29.5921) (-20.9073, -29.5992) (-20.9004, -29.6027) knots -1 -1 -1 -1 -1 -1 -0.98571429 -0.97142857 -0.95714286 -0.94285714 -0.92857143 -0.91428571 -0.9 -0.88571429 -0.87142857 -0.85714286 -0.84285714 -0.82857143 -0.81428571 -0.8 -0.78571429 -0.77142857 -0.75714286 -0.74285714 -0.72857143 -0.71428571 -0.7 -0.68571429 -0.67142857 -0.65714286 -0.64285714 -0.62857143 -0.61428571 -0.6 -0.58571429 -0.57142857 -0.55714286 -0.54285714 -0.52857143 -0.51428571 -0.5 -0.48571429 -0.47142857 -0.45714286 -0.44285714 -0.42857143 -0.41428571 -0.4 -0.38571429 -0.37142857 -0.35714286 -0.34285714 -0.32857143 -0.31428571 -0.3 -0.28571429 -0.27142857 -0.25714286 -0.24285714 -0.22857143 -0.21428571 -0.2 -0.18571429 -0.17142857 -0.15714286 -0.14285714 -0.12857143 -0.11428571 -0.1 -0.08571429 -0.07142857 -0.05714286 -0.04285714 -0.02857143 -0.01428571 0 0 0 0 0 0
  line L19 (-20.9004, -29.6027) -> (-19.6789, -30.2093)
  arc A39 (-19.4404, -30.8508) -> (-19.6789, -30.2093) centre (-19.9013, -30.6571) ccw
  circle A40 centre (-12.4806, -33.7751) radius 2.5
  line L20 (-9.981, -33.8193) -> (-14.9794, -33.698) construction
  line L21 (-9.981, -33.8193) -> (-14.4796, -33.7101) construction
  line L22 (-14.4796, -33.7101) -> (-14.5164, -35.2261)
  line L23 (-14.4796, -33.7101) -> (-14.4436, -32.2271)
  dimension "d63" = 4.5
  constraint coincident A40 L20.start
  constraint coincident A40 L20.end
  constraint parallel L20 L21
  constraint coincident A40 L22.end
  constraint perpendicular L21 L22
  constraint coincident A40 L23.end
  constraint perpendicular L20 L23
  measures "d63" distance of L20.start L21.end
extrude "Extrude3" add sketch "Sketch3 (6)" against normal blind 11.5 contours A40 L22 L23 picked at (-14.8088, -33.7131) sketch seen with x (1, 0, 0) y (0, 1, 0) z (0, 0, 1) at (-12.4806, -33.7751, 0.3316) bodies 4 in component "Spur Gear (10 teeth)"